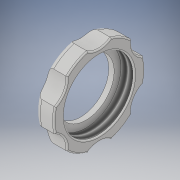
# Autodesk Inventor part: Крышка М
Saved by Autodesk Inventor 2019 (Build 230136000, 136)
## iProperties
Created: 2019-04-26
Part Number: Крышка М
Material: Типовые
Document SubType Name: Modeling
Designer: BarmanKaktus
Density: 1 g/cm^3
Appearance: По умолчанию
Author: BarmanKaktus
Autodesk Inventor part; units mm, degrees
ref_plane "XZ Plane" through (0, 0, 0) normal (0, 1, 0) x (-1, 0, 0)
ref_plane "XY Plane" through (0, 0, 0) normal (0, 0, 1) x (1, 0, 0)
sketch "Эскиз1" plane through (0, 0, 0) normal (0, 0, 1) x (1, 0, 0)
  line L0 (0, 0) -> (0, 30)
  line L1 (4, 34) -> (14, 34)
  line L2 (14, 34) -> (14, 26)
  line L3 (4, 0) -> (0, 0)
  arc A0 (4, 34) -> (0, 30) centre (4, 30) ccw
  line L4 (4, 0) -> (4, 26)
  line L5 (4, 26) -> (14, 26)
  dimension "d3" = 4
  dimension "d4" = 30
  dimension "d5" = 8
  dimension "d6" = 4
  dimension "d7" = 10
  dimension "d8" = 26
  constraints: 12 end point, 3 perpendicular, 2 point on circle, 2 tangent, 2 vertical, 1 centre point
  measures "d3" radius of A0
  measures "d4" distance of L0.start L0.end
  measures "d5" distance of L1.end L2.end
  measures "d6" distance of L3.start L0.start
  measures "d7" distance of L1.end L1.start
  measures "d8" distance of L3.start L4.end
revolve "Вращение1" add sketch "Эскиз1" angle 360 about axis through (4, 0, 0) along (-1, 0, 0)
ref_plane "РабПлоскость1" through (7, 0, 0) normal (1, 0, 0) x (0, 1, 0)
sketch "Эскиз4" plane through (7, 0, 0) normal (1, 0, 0) x (0, 1, 0)
  circle A0 centre (0, 0) radius 45
  circle A1 centre (45, 0) radius 15
  circle A2 centre (22.5, 38.9711) radius 15
  circle A3 centre (-22.5, 38.9711) radius 15
  circle A4 centre (-45, 0) radius 15
  circle A5 centre (-22.5, -38.9711) radius 15
  circle A6 centre (22.5, -38.9711) radius 15
  dimension "d10" = 90
  dimension "d11" = 30
  dimension "d14" = 360
  constraints: 6 centre point, 1 coincident, 1 horizontal alignment, 15 other
  measures "d11" diameter of A1
extrude "Выдавливание1" cut sketch "Эскиз4" along normal through all both and the other way through all contours A0 A1 | A0 A1 | A2 A0 | A0 A2 | A6 A0 | A0 A6 | A3 A0 | A0 A3 | A5 A0 | A0 A5 | A4 A0 | A0 A4
sketch "Эскиз5" plane through (7, 0, 0) normal (1, 0, 0) x (0, 1, 0)
  circle A0 centre (0, 0) radius 21
  dimension "d18" = 42
  constraints: 1 centre point, 1 coincident
  measures "d18" diameter of A0
extrude "Выдавливание2" cut sketch "Эскиз5" along normal through all both and the other way through all
thread "Резьба1" size "M52x5" class "6H" standard "ISO Metric profile" full length
thread "Резьба2" size "M52x5" class "6H" standard "ANSI Metric M Profile" full length
fillet "Сопряжение1" radius 1 13 edges at (14, 15, -25.9808) (14, 29.4449, -17) (14, 30, 0) (14, 29.4449, 17) (14, 15, 25.9808) (14, 0, 34) (14, -15, 25.9808) (14, -29.4449, 17) (14, -30, 0) (14, -29.4449, -17) (14, -15, -25.9808) (14, 0, -34) (14, -26, 0)
